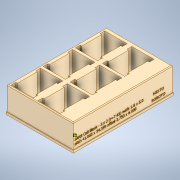
# Autodesk Inventor part: BlockTray_parameterized
Saved by Autodesk Inventor 2020 (Build 240168000, 168)
## iProperties
Created: 2019-12-05
Part Number: BlockTray_parameterized
Material: PC/ABS Plastic
Document SubType Name: Modeling
Designer: pab2
Density: 0.357273 g/cm^3
Appearance: Smooth - Off-White
Author: pab2
Autodesk Inventor part; units mm, degrees
(part 1 of 3)
ref_plane "YZ Plane" through (0, 0, 0) normal (1, 0, 0) x (0, 1, 0)
ref_plane "XZ Plane" through (0, 0, 0) normal (0, 1, 0) x (-1, 0, 0)
ref_plane "XY Plane" through (0, 0, 0) normal (0, 0, 1) x (1, 0, 0)
sketch "Sketch1" plane through (0, 0, 0) normal (0, 1, 0) x (-1, 0, 0)
  line L0 (0, 0) -> (-85.5, 0)
  line L1 (-85.5, 0) -> (-85.5, -127.75)
  line L2 (-85.5, -127.75) -> (0, -127.75)
  line L3 (0, -127.75) -> (0, 0)
  dimension "BaseW" = 85.5
  dimension "BaseL" = 127.75
  constraints: 8 end point, 2 parallel, 1 horizontal, 1 perpendicular
  measures "BaseW" distance of L2.end L1.end
  measures "BaseL" distance of L1.end L0.end
extrude "Extrusion1" add sketch "Sketch1" along normal blind 3
sketch "Sketch2" plane through (0, 3, 0) normal (0, 1, 0) x (1, 0, 0)
  line L0 (0, 127.75) -> (0, 0) projected
  line L1 (0, 0) -> (0.7071, 0.7071)
  line L2 (0, 0) -> (1, 0) construction
  line L3 (85.5, 127.75) -> (0, 127.75) projected
  line L4 (85.5, 127.75) -> (84.7929, 127.0429)
  line L5 (85.5, 127.75) -> (86.5, 127.75) construction
  line L6 (0.7071, 0.7071) -> (84.7929, 0.7071)
  line L7 (84.7929, 0.7071) -> (84.7929, 127.0429)
  line L8 (84.7929, 127.0429) -> (0.7071, 127.0429)
  line L9 (0.7071, 127.0429) -> (0.7071, 0.7071)
  dimension "RimOffset" = 1
  dimension "d5" = 45
  dimension "d6" = 1
  dimension "d7" = 225
  constraints: 16 end point, 3 horizontal, 2 equal length, 2 parallel, 1 perpendicular
  measures "RimOffset" distance of L0.end L1.end
  measures "d5" angle of L2 L1
  measures "d6" distance of L3.start L4.end
extrude "Extrusion2" add sketch "Sketch2" along normal blind 30 contours L9 L8 L7 L6
sketch "Sketch4" plane through (0, 33, 0) normal (0, 1, 0) x (1, 0, 0)
  line L0 (0.7071, 0.7071) -> (17.8022, 0.7071) construction
  line L1 (0.7071, 0.7071) -> (84.7929, 0.7071) projected
  line L2 (0.7071, 0.7071) -> (5.7071, 0.7071)
  line L3 (84.7929, 0.7071) -> (0.7071, 0.7071) projected
  line L4 (5.7071, 0.7071) -> (5.7071, 2.4571)
  line L5 (5.7071, 2.4571) -> (30.0657, 2.4571)
  line L6 (30.0657, 2.4571) -> (30.0657, 39.9602)
  line L7 (30.0657, 39.9602) -> (5.7071, 39.9602)
  line L8 (5.7071, 39.9602) -> (5.7071, 2.4571)
  line L9 (30.0657, 39.9602) -> (32.0657, 39.9602)
  line L10 (32.0657, 39.9602) -> (32.0657, 33.9602)
  line L11 (32.0657, 33.9602) -> (30.0657, 33.9602)
  line L12 (30.0657, 33.9602) -> (30.0657, 39.9602)
  line L13 (30.0657, 2.4571) -> (32.0657, 2.4571)
  line L14 (32.0657, 2.4571) -> (32.0657, 8.4571)
  line L15 (32.0657, 8.4571) -> (30.0657, 8.4571)
  line L16 (30.0657, 8.4571) -> (30.0657, 2.4571)
  line L17 (5.7071, 39.9602) -> (3.7071, 39.9602)
  line L18 (3.7071, 39.9602) -> (3.7071, 33.9602)
  line L19 (3.7071, 33.9602) -> (5.7071, 33.9602)
  line L20 (5.7071, 33.9602) -> (5.7071, 39.9602)
  line L21 (5.7071, 2.4571) -> (3.7071, 2.4571)
  line L22 (3.7071, 2.4571) -> (3.7071, 8.4571)
  line L23 (3.7071, 8.4571) -> (5.7071, 8.4571)
  line L24 (5.7071, 8.4571) -> (5.7071, 2.4571)
  point P0 (0, 0)
  point P1 (5.7071, 33.9602)
  point P2 (5.7071, 8.4571)
  point P3 (30.0657, 8.4571)
  dimension "d51" = 5
  dimension "d63" = 1.75
  dimension "d64" = 24.3586
  dimension "d65" = 37.5031
  dimension "ScrewProtrusionD" = 2
  dimension "ScrewProtrusionL" = 6
  dimension "d68" = 2
  dimension "d69" = 6
  dimension "d70" = 2
  dimension "d71" = 6
  dimension "d72" = 2
  dimension "d73" = 6
  constraints: 46 end point, 10 parallel, 6 horizontal, 6 perpendicular, 1 point on line
  measures "d51" distance of L0.start L2.end
  measures "d63" distance of L2.end L4.end
  measures "d64" distance of L7.end L6.end
  measures "d65" distance of L6.end L5.end
  measures "ScrewProtrusionD" distance of L10.end L11.end
  measures "ScrewProtrusionL" distance of L9.end L10.end
  measures "d68" distance of L15.end L14.end
  measures "d69" distance of L14.end L13.end
  measures "d70" distance of L19.end L18.end
  measures "d71" distance of L18.end L17.end
  measures "d72" distance of L22.end L23.end
  measures "d73" distance of L21.end L22.end
extrude "Extrusion3" cut sketch "Sketch4" against normal blind 30 from surface at 0
fillet "Fillet1" radius 1 4 edges at (42.75, 33, -0.7071) (84.7929, 33, -63.875) (0.7071, 33, -63.875) (42.75, 33, -127.0429)
pattern_linear "Rectangular Pattern2" count 2 spacing 34.3586 along (1, 0, 0) count 3 spacing 41.0031 along (0, 0, -1) of "Extrusion3"
sketch "Sketch5" plane through (84.7929, 3, -0.7071) normal (1, 0, 0) x (0, 0, -1)
  line L0 (1.5806, 11.976) -> (92.4463, 11.976) construction
  line L1 (92.4463, 11.976) -> (92.4463, 1.5433) construction
  line L2 (92.4463, 1.5433) -> (1.5806, 1.5433) construction
  line L3 (1.5806, 1.5433) -> (1.5806, 11.976) construction
  line L4 (95.1386, 13.0698) -> (121.8935, 13.0698) construction
  line L5 (121.8935, 13.0698) -> (121.8935, 1.4591) construction
  line L6 (121.8935, 1.4591) -> (95.1386, 1.4591) construction
  line L7 (95.1386, 1.4591) -> (95.1386, 13.0698) construction
  spline S0 degree 2 poles (2.7391, 8.7378) (2.4081, 8.7378) (1.9437, 8.8761) (1.7387, 8.9749) knots 0 0 0 1 2 2 2
  line L8 (1.7387, 8.9749) -> (1.7387, 9.4838)
  line L9 (1.7387, 9.4838) -> (1.7683, 9.4838)
  spline S1 degree 2 poles (1.7683, 9.4838) (1.9684, 9.296) (2.4748, 9.0886) (2.7094, 9.0886) knots 0 0 0 1 2 2 2
  spline S2 degree 2 poles (2.7094, 9.0886) (3.0453, 9.0886) (3.3887, 9.3677) (3.3887, 9.5974) knots 0 0 0 1 2 2 2
  spline S3 degree 2 poles (3.3887, 9.5974) (3.3887, 9.7802) (3.2084, 10.0074) (3.0132, 10.0642) knots 0 0 0 1 2 2 2
  spline S4 degree 2 poles (3.0132, 10.0642) (2.8724, 10.1037) (2.6378, 10.1581) (2.4624, 10.2025) knots 0 0 0 1 2 2 2
  spline S5 degree 2 poles (2.4624, 10.2025) (2.3043, 10.2445) (2.0549, 10.3705) (1.9585, 10.4718) knots 0 0 0 1 2 2 2
  spline S6 degree 2 poles (1.9585, 10.4718) (1.8647, 10.573) (1.7609, 10.8447) (1.7609, 11.0226) knots 0 0 0 1 2 2 2
  spline S7 degree 2 poles (1.7609, 11.0226) (1.7609, 11.3931) (2.3389, 11.8945) (2.786, 11.8945) knots 0 0 0 1 2 2 2
  spline S8 degree 2 poles (2.786, 11.8945) (3.0429, 11.8945) (3.4973, 11.7932) (3.6925, 11.6969) knots 0 0 0 1 2 2 2
  line L10 (3.6925, 11.6969) -> (3.6925, 11.2128)
  line L11 (3.6925, 11.2128) -> (3.6628, 11.2128)
  spline S9 degree 2 poles (3.6628, 11.2128) (3.5171, 11.3462) (3.0626, 11.5438) (2.8132, 11.5438) knots 0 0 0 1 2 2 2
  spline S10 degree 2 poles (2.8132, 11.5438) (2.5316, 11.5438) (2.1833, 11.2795) (2.1833, 11.0646) knots 0 0 0 1 2 2 2
  spline S11 degree 2 poles (2.1833, 11.0646) (2.1833, 10.8719) (2.3883, 10.6422) (2.581, 10.5903) knots 0 0 0 1 2 2 2
  spline S12 degree 2 poles (2.581, 10.5903) (2.7094, 10.5558) (3.0824, 10.4668) (3.2059, 10.4298) knots 0 0 0 1 2 2 2
  spline S13 degree 2 poles (3.2059, 10.4298) (3.5196, 10.3335) (3.811, 9.9457) (3.811, 9.6616) knots 0 0 0 1 2 2 2
  spline S14 degree 2 poles (3.811, 9.6616) (3.811, 9.4813) (3.6653, 9.1355) (3.5344, 9.0145) knots 0 0 0 1 2 2 2
  spline S15 degree 2 poles (3.5344, 9.0145) (3.3887, 8.8811) (3.0182, 8.7378) (2.7391, 8.7378) knots 0 0 0 1 2 2 2
  line L12 (3.895, 8.7922) -> (4.9225, 11.8402)
  line L13 (4.9225, 11.8402) -> (5.4215, 11.8402)
  line L14 (5.4215, 11.8402) -> (6.449, 8.7922)
  line L15 (6.449, 8.7922) -> (6.0217, 8.7922)
  line L16 (6.0217, 8.7922) -> (5.7451, 9.6443)
  line L17 (5.7451, 9.6443) -> (4.5817, 9.6443)
  line L18 (4.5817, 9.6443) -> (4.305, 8.7922)
  line L19 (4.305, 8.7922) -> (3.895, 8.7922)
  line L20 (5.6339, 9.9901) -> (5.1621, 11.4252)
  line L21 (5.1621, 11.4252) -> (4.6928, 9.9901)
  line L22 (4.6928, 9.9901) -> (5.6339, 9.9901)
  line L23 (8.919, 8.7922) -> (8.4646, 8.7922)
  line L24 (8.4646, 8.7922) -> (7.1159, 11.4203)
  line L25 (7.1159, 11.4203) -> (7.1159, 8.7922)
  line L26 (7.1159, 8.7922) -> (6.738, 8.7922)
  line L27 (6.738, 8.7922) -> (6.738, 11.8402)
  line L28 (6.738, 11.8402) -> (7.3135, 11.8402)
  line L29 (7.3135, 11.8402) -> (8.5411, 9.427)
  line L30 (8.5411, 9.427) -> (8.5411, 11.8402)
  line L31 (8.5411, 11.8402) -> (8.919, 11.8402)
  line L32 (8.919, 11.8402) -> (8.919, 8.7922)
  spline S16 degree 2 poles (10.3862, 8.7378) (10.0552, 8.7378) (9.5909, 8.8761) (9.3859, 8.9749) knots 0 0 0 1 2 2 2
  line L33 (9.3859, 8.9749) -> (9.3859, 9.4838)
  line L34 (9.3859, 9.4838) -> (9.4155, 9.4838)
  spline S17 degree 2 poles (9.4155, 9.4838) (9.6156, 9.296) (10.1219, 9.0886) (10.3566, 9.0886) knots 0 0 0 1 2 2 2
  spline S18 degree 2 poles (10.3566, 9.0886) (10.6925, 9.0886) (11.0358, 9.3677) (11.0358, 9.5974) knots 0 0 0 1 2 2 2
  spline S19 degree 2 poles (11.0358, 9.5974) (11.0358, 9.7802) (10.8555, 10.0074) (10.6604, 10.0642) knots 0 0 0 1 2 2 2
  spline S20 degree 2 poles (10.6604, 10.0642) (10.5196, 10.1037) (10.285, 10.1581) (10.1096, 10.2025) knots 0 0 0 1 2 2 2
  spline S21 degree 2 poles (10.1096, 10.2025) (9.9515, 10.2445) (9.702, 10.3705) (9.6057, 10.4718) knots 0 0 0 1 2 2 2
  spline S22 degree 2 poles (9.6057, 10.4718) (9.5118, 10.573) (9.4081, 10.8447) (9.4081, 11.0226) knots 0 0 0 1 2 2 2
  spline S23 degree 2 poles (9.4081, 11.0226) (9.4081, 11.3931) (9.9861, 11.8945) (10.4332, 11.8945) knots 0 0 0 1 2 2 2
  spline S24 degree 2 poles (10.4332, 11.8945) (10.69, 11.8945) (11.1445, 11.7932) (11.3396, 11.6969) knots 0 0 0 1 2 2 2
  line L35 (11.3396, 11.6969) -> (11.3396, 11.2128)
  line L36 (11.3396, 11.2128) -> (11.31, 11.2128)
  spline S25 degree 2 poles (11.31, 11.2128) (11.1643, 11.3462) (10.7098, 11.5438) (10.4603, 11.5438) knots 0 0 0 1 2 2 2
  spline S26 degree 2 poles (10.4603, 11.5438) (10.1787, 11.5438) (9.8305, 11.2795) (9.8305, 11.0646) knots 0 0 0 1 2 2 2
  spline S27 degree 2 poles (9.8305, 11.0646) (9.8305, 10.8719) (10.0355, 10.6422) (10.2281, 10.5903) knots 0 0 0 1 2 2 2
  spline S28 degree 2 poles (10.2281, 10.5903) (10.3566, 10.5558) (10.7296, 10.4668) (10.8531, 10.4298) knots 0 0 0 1 2 2 2
  spline S29 degree 2 poles (10.8531, 10.4298) (11.1667, 10.3335) (11.4582, 9.9457) (11.4582, 9.6616) knots 0 0 0 1 2 2 2
  spline S30 degree 2 poles (11.4582, 9.6616) (11.4582, 9.4813) (11.3125, 9.1355) (11.1816, 9.0145) knots 0 0 0 1 2 2 2
  spline S31 degree 2 poles (11.1816, 9.0145) (11.0358, 8.8811) (10.6653, 8.7378) (10.3862, 8.7378) knots 0 0 0 1 2 2 2
  spline S32 degree 2 poles (14.3704, 8.7378) (14.074, 8.7378) (13.5725, 8.9379) (13.3898, 9.138) knots 0 0 0 1 2 2 2
  spline S33 degree 2 poles (13.3898, 9.138) (13.207, 9.3356) (13.0069, 9.9284) (13.0069, 10.3137) knots 0 0 0 1 2 2 2
  spline S34 degree 2 poles (13.0069, 10.3137) (13.0069, 10.6965) (13.202, 11.2646) (13.3873, 11.4746) knots 0 0 0 1 2 2 2
  spline S35 degree 2 poles (13.3873, 11.4746) (13.5701, 11.6796) (14.069, 11.8945) (14.3778, 11.8945) knots 0 0 0 1 2 2 2
  spline S36 degree 2 poles (14.3778, 11.8945) (14.5309, 11.8945) (14.8001, 11.85) (14.9138, 11.8155) knots 0 0 0 1 2 2 2
  spline S37 degree 2 poles (14.9138, 11.8155) (15.0126, 11.7834) (15.2176, 11.692) (15.3188, 11.6376) knots 0 0 0 1 2 2 2
  line L37 (15.3188, 11.6376) -> (15.3188, 11.1486)
  line L38 (15.3188, 11.1486) -> (15.2867, 11.1486)
  spline S38 degree 2 poles (15.2867, 11.1486) (15.2324, 11.198) (15.0644, 11.3363) (14.9434, 11.403) knots 0 0 0 1 2 2 2
  spline S39 degree 2 poles (14.9434, 11.403) (14.8273, 11.4672) (14.5531, 11.5487) (14.3753, 11.5487) knots 0 0 0 1 2 2 2
  spline S40 degree 2 poles (14.3753, 11.5487) (14.1802, 11.5487) (13.8319, 11.3881) (13.701, 11.235) knots 0 0 0 1 2 2 2
  spline S41 degree 2 poles (13.701, 11.235) (13.5725, 11.0794) (13.4293, 10.6076) (13.4293, 10.3137) knots 0 0 0 1 2 2 2
  spline S42 degree 2 poles (13.4293, 10.3137) (13.4293, 10) (13.58, 9.548) (13.7109, 9.3924) knots 0 0 0 1 2 2 2
  spline S43 degree 2 poles (13.7109, 9.3924) (13.8393, 9.2417) (14.1826, 9.0886) (14.3753, 9.0886) knots 0 0 0 1 2 2 2
  spline S44 degree 2 poles (14.3753, 9.0886) (14.5507, 9.0886) (14.8495, 9.175) (14.9656, 9.2392) knots 0 0 0 1 2 2 2
  spline S45 degree 2 poles (14.9656, 9.2392) (15.0768, 9.3035) (15.2423, 9.4368) (15.2892, 9.4838) knots 0 0 0 1 2 2 2
  line L39 (15.2892, 9.4838) -> (15.3188, 9.4838)
  line L40 (15.3188, 9.4838) -> (15.3188, 8.9996)
  spline S46 degree 2 poles (15.3188, 8.9996) (15.2176, 8.9527) (15.0397, 8.8663) (14.9138, 8.8267) knots 0 0 0 1 2 2 2
  spline S47 degree 2 poles (14.9138, 8.8267) (14.7804, 8.7823) (14.5531, 8.7378) (14.3704, 8.7378) knots 0 0 0 1 2 2 2
  spline S48 degree 2 poles (16.6601, 8.7403) (16.1117, 8.7403) (15.509, 9.3553) (15.509, 9.9234) knots 0 0 0 1 2 2 2
  spline S49 degree 2 poles (15.509, 9.9234) (15.509, 10.4817) (16.0944, 11.1436) (16.5662, 11.1436) knots 0 0 0 1 2 2 2
  spline S50 degree 2 poles (16.5662, 11.1436) (16.7786, 11.1436) (17.1071, 11.0201) (17.2282, 10.8892) knots 0 0 0 1 2 2 2
  spline S51 degree 2 poles (17.2282, 10.8892) (17.3517, 10.7583) (17.4826, 10.3804) (17.4826, 10.1062) knots 0 0 0 1 2 2 2
  line L41 (17.4826, 10.1062) -> (17.4826, 9.8963)
  line L42 (17.4826, 9.8963) -> (15.8993, 9.8963)
  spline S52 degree 2 poles (15.8993, 9.8963) (15.8993, 9.4986) (16.2994, 9.0762) (16.6551, 9.0762) knots 0 0 0 1 2 2 2
  spline S53 degree 2 poles (16.6551, 9.0762) (16.7811, 9.0762) (17.0256, 9.133) (17.1244, 9.1775) knots 0 0 0 1 2 2 2
  spline S54 degree 2 poles (17.1244, 9.1775) (17.2282, 9.2269) (17.3714, 9.3133) (17.4184, 9.3529) knots 0 0 0 1 2 2 2
  line L43 (17.4184, 9.3529) -> (17.4406, 9.3529)
  line L44 (17.4406, 9.3529) -> (17.4406, 8.933)
  spline S55 degree 2 poles (17.4406, 8.933) (17.3739, 8.9058) (17.1714, 8.8267) (17.0923, 8.8045) knots 0 0 0 1 2 2 2
  spline S56 degree 2 poles (17.0923, 8.8045) (16.9812, 8.7724) (16.7984, 8.7403) (16.6601, 8.7403) knots 0 0 0 1 2 2 2
  spline S57 degree 2 poles (17.1071, 10.1902) (17.1022, 10.3458) (17.038, 10.573) (16.9762, 10.6496) knots 0 0 0 1 2 2 2
  spline S58 degree 2 poles (16.9762, 10.6496) (16.9095, 10.7361) (16.6996, 10.8275) (16.544, 10.8275) knots 0 0 0 1 2 2 2
  spline S59 degree 2 poles (16.544, 10.8275) (16.3908, 10.8275) (16.1759, 10.7361) (16.087, 10.6471) knots 0 0 0 1 2 2 2
  spline S60 degree 2 poles (16.087, 10.6471) (16.0006, 10.5558) (15.9116, 10.3359) (15.8993, 10.1902) knots 0 0 0 1 2 2 2
  line L45 (15.8993, 10.1902) -> (17.1071, 10.1902)
  line L46 (18.2656, 8.7922) -> (17.8803, 8.7922)
  line L47 (17.8803, 8.7922) -> (17.8803, 11.976)
  line L48 (17.8803, 11.976) -> (18.2656, 11.976)
  line L49 (18.2656, 11.976) -> (18.2656, 8.7922)
  line L50 (19.2239, 8.7922) -> (18.8386, 8.7922)
  line L51 (18.8386, 8.7922) -> (18.8386, 11.976)
  line L52 (18.8386, 11.976) -> (19.2239, 11.976)
  line L53 (19.2239, 11.976) -> (19.2239, 8.7922)
  spline S61 degree 2 poles (23.1957, 9.7283) (23.1957, 9.5011) (23.0228, 9.1528) (22.8796, 9.0392) knots 0 0 0 1 2 2 2
  spline S62 degree 2 poles (22.8796, 9.0392) (22.7067, 8.9058) (22.3139, 8.7922) (22.0027, 8.7922) knots 0 0 0 1 2 2 2
  line L54 (22.0027, 8.7922) -> (21.1283, 8.7922)
  line L55 (21.1283, 8.7922) -> (21.1283, 11.8402)
  line L56 (21.1283, 11.8402) -> (21.936, 11.8402)
  spline S63 degree 2 poles (21.936, 11.8402) (22.2621, 11.8402) (22.5881, 11.7982) (22.7363, 11.7167) knots 0 0 0 1 2 2 2
  spline S64 degree 2 poles (22.7363, 11.7167) (22.9018, 11.6302) (23.0525, 11.3462) (23.0525, 11.1535) knots 0 0 0 1 2 2 2
  spline S65 degree 2 poles (23.0525, 11.1535) (23.0525, 10.9386) (22.8252, 10.5977) (22.6252, 10.5014) knots 0 0 0 1 2 2 2
  line L57 (22.6252, 10.5014) -> (22.6252, 10.4866)
  spline S66 degree 2 poles (22.6252, 10.4866) (22.8969, 10.4125) (23.1957, 10.0198) (23.1957, 9.7283) knots 0 0 0 1 2 2 2
  spline S67 degree 2 poles (22.7734, 9.711) (22.7734, 9.8839) (22.6746, 10.1062) (22.5264, 10.1853) knots 0 0 0 1 2 2 2
  spline S68 degree 2 poles (22.5264, 10.1853) (22.43, 10.2347) (22.2028, 10.2643) (21.9928, 10.2643) knots 0 0 0 1 2 2 2
  line L58 (21.9928, 10.2643) -> (21.5334, 10.2643)
  line L59 (21.5334, 10.2643) -> (21.5334, 9.138)
  line L60 (21.5334, 9.138) -> (21.8619, 9.138)
  spline S69 degree 2 poles (21.8619, 9.138) (22.1287, 9.138) (22.435, 9.1874) (22.5535, 9.2664) knots 0 0 0 1 2 2 2
  spline S70 degree 2 poles (22.5535, 9.2664) (22.6671, 9.3479) (22.7734, 9.5505) (22.7734, 9.711) knots 0 0 0 1 2 2 2
  spline S71 degree 2 poles (22.6301, 11.0967) (22.6301, 11.2054) (22.556, 11.3684) (22.4745, 11.4153) knots 0 0 0 1 2 2 2
  spline S72 degree 2 poles (22.4745, 11.4153) (22.3757, 11.4697) (22.1361, 11.4944) (21.9212, 11.4944) knots 0 0 0 1 2 2 2
  line L61 (21.9212, 11.4944) -> (21.5334, 11.4944)
  line L62 (21.5334, 11.4944) -> (21.5334, 10.6027)
  line L63 (21.5334, 10.6027) -> (21.9928, 10.6027)
  spline S73 degree 2 poles (21.9928, 10.6027) (22.183, 10.6027) (22.3633, 10.6422) (22.4597, 10.704) knots 0 0 0 1 2 2 2
  spline S74 degree 2 poles (22.4597, 10.704) (22.5535, 10.7632) (22.6301, 10.9534) (22.6301, 11.0967) knots 0 0 0 1 2 2 2
  line L64 (23.9614, 8.7922) -> (23.5761, 8.7922)
  line L65 (23.5761, 8.7922) -> (23.5761, 11.976)
  line L66 (23.5761, 11.976) -> (23.9614, 11.976)
  line L67 (23.9614, 11.976) -> (23.9614, 8.7922)
  spline S75 degree 2 poles (26.4067, 9.9358) (26.4067, 9.3578) (25.851, 8.7279) (25.3866, 8.7279) knots 0 0 0 1 2 2 2
  spline S76 degree 2 poles (25.3866, 8.7279) (24.9099, 8.7279) (24.364, 9.3776) (24.364, 9.9358) knots 0 0 0 1 2 2 2
  spline S77 degree 2 poles (24.364, 9.9358) (24.364, 10.5088) (24.9272, 11.1436) (25.3866, 11.1436) knots 0 0 0 1 2 2 2
  spline S78 degree 2 poles (25.3866, 11.1436) (25.851, 11.1436) (26.4067, 10.5113) (26.4067, 9.9358) knots 0 0 0 1 2 2 2
  spline S79 degree 2 poles (26.0091, 9.9358) (26.0091, 10.3804) (25.6855, 10.8126) (25.3866, 10.8126) knots 0 0 0 1 2 2 2
  spline S80 degree 2 poles (25.3866, 10.8126) (25.0878, 10.8126) (24.7617, 10.3804) (24.7617, 9.9358) knots 0 0 0 1 2 2 2
  spline S81 degree 2 poles (24.7617, 9.9358) (24.7617, 9.5035) (25.0878, 9.0589) (25.3866, 9.0589) knots 0 0 0 1 2 2 2
  spline S82 degree 2 poles (25.3866, 9.0589) (25.683, 9.0589) (26.0091, 9.4961) (26.0091, 9.9358) knots 0 0 0 1 2 2 2
  spline S83 degree 2 poles (27.7109, 8.7403) (27.4738, 8.7403) (27.0811, 8.886) (26.9403, 9.0342) knots 0 0 0 1 2 2 2
  spline S84 degree 2 poles (26.9403, 9.0342) (26.7995, 9.18) (26.6439, 9.6295) (26.6439, 9.9308) knots 0 0 0 1 2 2 2
  spline S85 degree 2 poles (26.6439, 9.9308) (26.6439, 10.2322) (26.8044, 10.6718) (26.9403, 10.82) knots 0 0 0 1 2 2 2
  spline S86 degree 2 poles (26.9403, 10.82) (27.0761, 10.9707) (27.4787, 11.1313) (27.7109, 11.1313) knots 0 0 0 1 2 2 2
  spline S87 degree 2 poles (27.7109, 11.1313) (27.8986, 11.1313) (28.2494, 11.0251) (28.3852, 10.9559) knots 0 0 0 1 2 2 2
  line L68 (28.3852, 10.9559) -> (28.3852, 10.5236)
  line L69 (28.3852, 10.5236) -> (28.363, 10.5236)
  spline S88 degree 2 poles (28.363, 10.5236) (28.321, 10.5582) (28.1926, 10.6471) (28.1012, 10.6941) knots 0 0 0 1 2 2 2
  spline S89 degree 2 poles (28.1012, 10.6941) (28.0197, 10.7336) (27.8023, 10.7953) (27.7035, 10.7953) knots 0 0 0 1 2 2 2
  spline S90 degree 2 poles (27.7035, 10.7953) (27.4046, 10.7953) (27.0415, 10.3433) (27.0415, 9.9308) knots 0 0 0 1 2 2 2
  spline S91 degree 2 poles (27.0415, 9.9308) (27.0415, 9.5282) (27.3923, 9.0762) (27.7035, 9.0762) knots 0 0 0 1 2 2 2
  spline S92 degree 2 poles (27.7035, 9.0762) (27.8912, 9.0762) (28.2321, 9.2318) (28.363, 9.3529) knots 0 0 0 1 2 2 2
  line L70 (28.363, 9.3529) -> (28.3852, 9.3529)
  line L71 (28.3852, 9.3529) -> (28.3852, 8.9206)
  spline S93 degree 2 poles (28.3852, 8.9206) (28.3284, 8.8934) (28.1555, 8.8169) (28.0864, 8.7996) knots 0 0 0 1 2 2 2
  spline S94 degree 2 poles (28.0864, 8.7996) (27.9876, 8.7699) (27.8319, 8.7403) (27.7109, 8.7403) knots 0 0 0 1 2 2 2
  line L72 (30.6305, 8.7922) -> (30.1241, 8.7922)
  line L73 (30.1241, 8.7922) -> (29.2744, 9.8963)
  line L74 (29.2744, 9.8963) -> (29.1213, 9.7481)
  line L75 (29.1213, 9.7481) -> (29.1213, 8.7922)
  line L76 (29.1213, 8.7922) -> (28.736, 8.7922)
  line L77 (28.736, 8.7922) -> (28.736, 11.976)
  line L78 (28.736, 11.976) -> (29.1213, 11.976)
  line L79 (29.1213, 11.976) -> (29.1213, 10.1136)
  line L80 (29.1213, 10.1136) -> (30.0253, 11.0794)
  line L81 (30.0253, 11.0794) -> (30.5045, 11.0794)
  line L82 (30.5045, 11.0794) -> (29.5659, 10.1235)
  line L83 (29.5659, 10.1235) -> (30.6305, 8.7922)
  line L84 (33.1919, 9.9407) -> (32.0384, 9.9407)
  line L85 (32.0384, 9.9407) -> (32.0384, 10.3112)
  line L86 (32.0384, 10.3112) -> (33.1919, 10.3112)
  line L87 (33.1919, 10.3112) -> (33.1919, 9.9407)
  spline S95 degree 2 poles (35.7286, 11.5512) (35.6174, 11.5512) (35.3976, 11.4968) (35.2914, 11.4548) knots 0 0 0 1 2 2 2
  spline S96 degree 2 poles (35.2914, 11.4548) (35.1926, 11.4128) (35.0469, 11.3239) (34.9901, 11.2844) knots 0 0 0 1 2 2 2
  line L88 (34.9901, 11.2844) -> (34.9654, 11.2844)
  line L89 (34.9654, 11.2844) -> (34.9654, 11.7167)
  spline S97 degree 2 poles (34.9654, 11.7167) (35.0987, 11.7883) (35.5557, 11.9044) (35.7607, 11.9044) knots 0 0 0 1 2 2 2
  spline S98 degree 2 poles (35.7607, 11.9044) (35.9682, 11.9044) (36.2769, 11.8204) (36.4029, 11.7315) knots 0 0 0 1 2 2 2
  spline S99 degree 2 poles (36.4029, 11.7315) (36.5363, 11.6351) (36.6746, 11.356) (36.6746, 11.1683) knots 0 0 0 1 2 2 2
  spline S100 degree 2 poles (36.6746, 11.1683) (36.6746, 10.9164) (36.3436, 10.536) (36.1114, 10.4866) knots 0 0 0 1 2 2 2
  line L90 (36.1114, 10.4866) -> (36.1114, 10.457)
  spline S101 degree 2 poles (36.1114, 10.457) (36.2078, 10.4372) (36.4276, 10.3483) (36.5215, 10.2594) knots 0 0 0 1 2 2 2
  spline S102 degree 2 poles (36.5215, 10.2594) (36.6153, 10.1729) (36.7339, 9.8963) (36.7339, 9.6962) knots 0 0 0 1 2 2 2
  spline S103 degree 2 poles (36.7339, 9.6962) (36.7339, 9.4912) (36.5931, 9.1429) (36.4647, 9.0095) knots 0 0 0 1 2 2 2
  spline S104 degree 2 poles (36.4647, 9.0095) (36.3313, 8.8712) (35.9534, 8.7279) (35.7138, 8.7279) knots 0 0 0 1 2 2 2
  spline S105 degree 2 poles (35.7138, 8.7279) (35.4841, 8.7279) (35.0345, 8.8391) (34.8814, 8.9157) knots 0 0 0 1 2 2 2
  line L91 (34.8814, 8.9157) -> (34.8814, 9.3479)
  line L92 (34.8814, 9.3479) -> (34.911, 9.3479)
  spline S106 degree 2 poles (34.911, 9.3479) (35.0395, 9.2541) (35.4742, 9.0812) (35.6891, 9.0812) knots 0 0 0 1 2 2 2
  spline S107 degree 2 poles (35.6891, 9.0812) (35.815, 9.0812) (36.067, 9.1602) (36.151, 9.2516) knots 0 0 0 1 2 2 2
  spline S108 degree 2 poles (36.151, 9.2516) (36.2325, 9.343) (36.3189, 9.5603) (36.3189, 9.7258) knots 0 0 0 1 2 2 2
  spline S109 degree 2 poles (36.3189, 9.7258) (36.3189, 9.8913) (36.2226, 10.1062) (36.1361, 10.168) knots 0 0 0 1 2 2 2
  spline S110 degree 2 poles (36.1361, 10.168) (36.0497, 10.2297) (35.815, 10.2766) (35.6767, 10.2766) knots 0 0 0 1 2 2 2
  line L93 (35.6767, 10.2766) -> (35.5038, 10.2766)
  line L94 (35.5038, 10.2766) -> (35.5038, 10.615)
  line L95 (35.5038, 10.615) -> (35.6397, 10.615)
  spline S111 degree 2 poles (35.6397, 10.615) (35.9138, 10.615) (36.2596, 10.8769) (36.2596, 11.1263) knots 0 0 0 1 2 2 2
  spline S112 degree 2 poles (36.2596, 11.1263) (36.2596, 11.2424) (36.1707, 11.4079) (36.0991, 11.4573) knots 0 0 0 1 2 2 2
  spline S113 degree 2 poles (36.0991, 11.4573) (36.0225, 11.5092) (35.8348, 11.5512) (35.7286, 11.5512) knots 0 0 0 1 2 2 2
  line L96 (40.3352, 8.7922) -> (39.8634, 8.7922)
  line L97 (39.8634, 8.7922) -> (39.3076, 9.6517)
  line L98 (39.3076, 9.6517) -> (38.7371, 8.7922)
  line L99 (38.7371, 8.7922) -> (38.2999, 8.7922)
  line L100 (38.2999, 8.7922) -> (39.0928, 9.9259)
  line L101 (39.0928, 9.9259) -> (38.3073, 11.0794)
  line L102 (38.3073, 11.0794) -> (38.7791, 11.0794)
  line L103 (38.7791, 11.0794) -> (39.3323, 10.2272)
  line L104 (39.3323, 10.2272) -> (39.898, 11.0794)
  line L105 (39.898, 11.0794) -> (40.3352, 11.0794)
  line L106 (40.3352, 11.0794) -> (39.5472, 9.9506)
  line L107 (39.5472, 9.9506) -> (40.3352, 8.7922)
  line L108 (43.766, 8.7922) -> (41.8863, 8.7922)
  line L109 (41.8863, 8.7922) -> (41.8863, 9.2244)
  spline S114 degree 2 poles (41.8863, 9.2244) (42.0889, 9.4146) (42.4495, 9.7678) (42.6224, 9.958) knots 0 0 0 1 2 2 2
  spline S115 degree 2 poles (42.6224, 9.958) (42.9707, 10.3409) (43.2251, 10.8003) (43.2251, 11.0448) knots 0 0 0 1 2 2 2
  spline S116 degree 2 poles (43.2251, 11.0448) (43.2251, 11.1733) (43.146, 11.3659) (43.0744, 11.4277) knots 0 0 0 1 2 2 2
  spline S117 degree 2 poles (43.0744, 11.4277) (43.0028, 11.4894) (42.8151, 11.5512) (42.7014, 11.5512) knots 0 0 0 1 2 2 2
  spline S118 degree 2 poles (42.7014, 11.5512) (42.5928, 11.5512) (42.3705, 11.4968) (42.2692, 11.4548) knots 0 0 0 1 2 2 2
  spline S119 degree 2 poles (42.2692, 11.4548) (42.1827, 11.4203) (42.0222, 11.3215) (41.9728, 11.2869) knots 0 0 0 1 2 2 2
  line L110 (41.9728, 11.2869) -> (41.9506, 11.2869)
  line L111 (41.9506, 11.2869) -> (41.9506, 11.7216)
  spline S120 degree 2 poles (41.9506, 11.7216) (42.0765, 11.7834) (42.5285, 11.9044) (42.7311, 11.9044) knots 0 0 0 1 2 2 2
  spline S121 degree 2 poles (42.7311, 11.9044) (43.1584, 11.9044) (43.6401, 11.4524) (43.6401, 11.067) knots 0 0 0 1 2 2 2
  spline S122 degree 2 poles (43.6401, 11.067) (43.6401, 10.8867) (43.5561, 10.5854) (43.482, 10.457) knots 0 0 0 1 2 2 2
  spline S123 degree 2 poles (43.482, 10.457) (43.4079, 10.3236) (43.193, 10.0617) (43.0744, 9.9358) knots 0 0 0 1 2 2 2
  spline S124 degree 2 poles (43.0744, 9.9358) (42.8818, 9.7258) (42.41, 9.2763) (42.2692, 9.1454) knots 0 0 0 1 2 2 2
  line L112 (42.2692, 9.1454) -> (43.766, 9.1454)
  line L113 (43.766, 9.1454) -> (43.766, 8.7922)
  line L114 (46.7128, 7.9499) -> (46.2434, 7.9499)
  spline S125 degree 2 poles (46.2434, 7.9499) (45.8878, 8.3723) (45.4802, 9.3183) (45.4802, 9.9629) knots 0 0 0 1 2 2 2
  spline S126 degree 2 poles (45.4802, 9.9629) (45.4802, 10.5928) (45.8828, 11.5536) (46.2434, 11.976) knots 0 0 0 1 2 2 2
  line L115 (46.2434, 11.976) -> (46.7128, 11.976)
  line L116 (46.7128, 11.976) -> (46.7128, 11.9563)
  spline S127 degree 2 poles (46.7128, 11.9563) (46.5473, 11.8056) (46.2459, 11.4153) (46.1175, 11.156) knots 0 0 0 1 2 2 2
  spline S128 degree 2 poles (46.1175, 11.156) (45.994, 10.904) (45.8408, 10.2989) (45.8408, 9.9629) knots 0 0 0 1 2 2 2
  spline S129 degree 2 poles (45.8408, 9.9629) (45.8408, 9.6122) (45.989, 9.0318) (46.1175, 8.7699) knots 0 0 0 1 2 2 2
  spline S130 degree 2 poles (46.1175, 8.7699) (46.241, 8.518) (46.5547, 8.1104) (46.7128, 7.9696) knots 0 0 0 1 2 2 2
  line L117 (46.7128, 7.9696) -> (46.7128, 7.9499)
  line L118 (48.3578, 10.6669) -> (48.338, 10.6669)
  spline S131 degree 2 poles (48.338, 10.6669) (48.2936, 10.6793) (48.1972, 10.6842) (48.1305, 10.6842) knots 0 0 0 1 2 2 2
  spline S132 degree 2 poles (48.1305, 10.6842) (47.9749, 10.6842) (47.6686, 10.5483) (47.5303, 10.415) knots 0 0 0 1 2 2 2
  line L119 (47.5303, 10.415) -> (47.5303, 8.7922)
  line L120 (47.5303, 8.7922) -> (47.145, 8.7922)
  line L121 (47.145, 8.7922) -> (47.145, 11.0794)
  line L122 (47.145, 11.0794) -> (47.5303, 11.0794)
  line L123 (47.5303, 11.0794) -> (47.5303, 10.7385)
  spline S133 degree 2 poles (47.5303, 10.7385) (47.7403, 10.9263) (48.054, 11.0794) (48.2022, 11.0794) knots 0 0 0 1 2 2 2
  spline S134 degree 2 poles (48.2022, 11.0794) (48.2615, 11.0794) (48.3207, 11.0745) (48.3578, 11.067) knots 0 0 0 1 2 2 2
  line L124 (48.3578, 11.067) -> (48.3578, 10.6669)
  line L125 (51.0328, 9.5332) -> (48.7703, 9.5332)
  line L126 (48.7703, 9.5332) -> (48.7703, 9.8617)
  line L127 (48.7703, 9.8617) -> (51.0328, 9.8617)
  line L128 (51.0328, 9.8617) -> (51.0328, 9.5332)
  line L129 (51.0328, 10.3927) -> (48.7703, 10.3927)
  line L130 (48.7703, 10.3927) -> (48.7703, 10.7212)
  line L131 (48.7703, 10.7212) -> (51.0328, 10.7212)
  line L132 (51.0328, 10.7212) -> (51.0328, 10.3927)
  line L133 (53.5646, 11.3832) -> (52.2456, 8.7922)
  line L134 (52.2456, 8.7922) -> (51.8109, 8.7922)
  line L135 (51.8109, 8.7922) -> (53.204, 11.482)
  line L136 (53.204, 11.482) -> (51.6306, 11.482)
  line L137 (51.6306, 11.482) -> (51.6306, 11.8402)
  line L138 (51.6306, 11.8402) -> (53.5646, 11.8402)
  line L139 (53.5646, 11.8402) -> (53.5646, 11.3832)
  line L140 (54.5921, 8.7922) -> (54.103, 8.7922)
  line L141 (54.103, 8.7922) -> (54.103, 9.3751)
  line L142 (54.103, 9.3751) -> (54.5921, 9.3751)
  line L143 (54.5921, 9.3751) -> (54.5921, 8.7922)
  line L144 (57.1683, 9.8394) -> (56.8052, 9.8394)
  line L145 (56.8052, 9.8394) -> (56.8052, 8.7922)
  line L146 (56.8052, 8.7922) -> (56.4125, 8.7922)
  line L147 (56.4125, 8.7922) -> (56.4125, 9.8394)
  line L148 (56.4125, 9.8394) -> (55.0663, 9.8394)
  line L149 (55.0663, 9.8394) -> (55.0663, 10.2692)
  line L150 (55.0663, 10.2692) -> (56.4298, 11.8402)
  line L151 (56.4298, 11.8402) -> (56.8052, 11.8402)
  line L152 (56.8052, 11.8402) -> (56.8052, 10.168)
  line L153 (56.8052, 10.168) -> (57.1683, 10.168)
  line L154 (57.1683, 10.168) -> (57.1683, 9.8394)
  line L155 (56.4125, 10.168) -> (56.4125, 11.3585)
  line L156 (56.4125, 11.3585) -> (55.3874, 10.168)
  line L157 (55.3874, 10.168) -> (56.4125, 10.168)
  spline S135 degree 2 poles (58.3169, 11.5512) (58.2057, 11.5512) (57.9859, 11.4968) (57.8797, 11.4548) knots 0 0 0 1 2 2 2
  spline S136 degree 2 poles (57.8797, 11.4548) (57.7809, 11.4128) (57.6352, 11.3239) (57.5784, 11.2844) knots 0 0 0 1 2 2 2
  line L158 (57.5784, 11.2844) -> (57.5537, 11.2844)
  line L159 (57.5537, 11.2844) -> (57.5537, 11.7167)
  spline S137 degree 2 poles (57.5537, 11.7167) (57.687, 11.7883) (58.144, 11.9044) (58.349, 11.9044) knots 0 0 0 1 2 2 2
  spline S138 degree 2 poles (58.349, 11.9044) (58.5565, 11.9044) (58.8652, 11.8204) (58.9912, 11.7315) knots 0 0 0 1 2 2 2
  spline S139 degree 2 poles (58.9912, 11.7315) (59.1246, 11.6351) (59.2629, 11.356) (59.2629, 11.1683) knots 0 0 0 1 2 2 2
  spline S140 degree 2 poles (59.2629, 11.1683) (59.2629, 10.9164) (58.9319, 10.536) (58.6997, 10.4866) knots 0 0 0 1 2 2 2
  line L160 (58.6997, 10.4866) -> (58.6997, 10.457)
  spline S141 degree 2 poles (58.6997, 10.457) (58.7961, 10.4372) (59.0159, 10.3483) (59.1098, 10.2594) knots 0 0 0 1 2 2 2
  spline S142 degree 2 poles (59.1098, 10.2594) (59.2036, 10.1729) (59.3222, 9.8963) (59.3222, 9.6962) knots 0 0 0 1 2 2 2
  spline S143 degree 2 poles (59.3222, 9.6962) (59.3222, 9.4912) (59.1814, 9.1429) (59.053, 9.0095) knots 0 0 0 1 2 2 2
  spline S144 degree 2 poles (59.053, 9.0095) (58.9196, 8.8712) (58.5417, 8.7279) (58.3021, 8.7279) knots 0 0 0 1 2 2 2
  spline S145 degree 2 poles (58.3021, 8.7279) (58.0724, 8.7279) (57.6228, 8.8391) (57.4697, 8.9157) knots 0 0 0 1 2 2 2
  line L161 (57.4697, 8.9157) -> (57.4697, 9.3479)
  line L162 (57.4697, 9.3479) -> (57.4993, 9.3479)
  spline S146 degree 2 poles (57.4993, 9.3479) (57.6278, 9.2541) (58.0625, 9.0812) (58.2774, 9.0812) knots 0 0 0 1 2 2 2
  spline S147 degree 2 poles (58.2774, 9.0812) (58.4033, 9.0812) (58.6553, 9.1602) (58.7393, 9.2516) knots 0 0 0 1 2 2 2
  spline S148 degree 2 poles (58.7393, 9.2516) (58.8208, 9.343) (58.9072, 9.5603) (58.9072, 9.7258) knots 0 0 0 1 2 2 2
  spline S149 degree 2 poles (58.9072, 9.7258) (58.9072, 9.8913) (58.8109, 10.1062) (58.7244, 10.168) knots 0 0 0 1 2 2 2
  spline S150 degree 2 poles (58.7244, 10.168) (58.638, 10.2297) (58.4033, 10.2766) (58.265, 10.2766) knots 0 0 0 1 2 2 2
  line L163 (58.265, 10.2766) -> (58.0921, 10.2766)
  line L164 (58.0921, 10.2766) -> (58.0921, 10.615)
  line L165 (58.0921, 10.615) -> (58.228, 10.615)
  spline S151 degree 2 poles (58.228, 10.615) (58.5021, 10.615) (58.8479, 10.8769) (58.8479, 11.1263) knots 0 0 0 1 2 2 2
  spline S152 degree 2 poles (58.8479, 11.1263) (58.8479, 11.2424) (58.759, 11.4079) (58.6874, 11.4573) knots 0 0 0 1 2 2 2
  spline S153 degree 2 poles (58.6874, 11.4573) (58.6108, 11.5092) (58.4231, 11.5512) (58.3169, 11.5512) knots 0 0 0 1 2 2 2
  spline S154 degree 2 poles (60.945, 9.9629) (60.945, 9.3306) (60.5399, 8.3723) (60.1818, 7.9499) knots 0 0 0 1 2 2 2
  line L166 (60.1818, 7.9499) -> (59.7124, 7.9499)
  line L167 (59.7124, 7.9499) -> (59.7124, 7.9696)
  spline S155 degree 2 poles (59.7124, 7.9696) (59.8705, 8.1104) (60.1892, 8.5229) (60.3077, 8.7699) knots 0 0 0 1 2 2 2
  spline S156 degree 2 poles (60.3077, 8.7699) (60.4362, 9.0342) (60.5844, 9.6221) (60.5844, 9.9629) knots 0 0 0 1 2 2 2
  spline S157 degree 2 poles (60.5844, 9.9629) (60.5844, 10.3013) (60.4337, 10.9016) (60.3077, 11.156) knots 0 0 0 1 2 2 2
  spline S158 degree 2 poles (60.3077, 11.156) (60.1842, 11.4104) (59.8681, 11.8155) (59.7124, 11.9563) knots 0 0 0 1 2 2 2
  line L168 (59.7124, 11.9563) -> (59.7124, 11.976)
  line L169 (59.7124, 11.976) -> (60.1818, 11.976)
  spline S159 degree 2 poles (60.1818, 11.976) (60.5374, 11.5536) (60.945, 10.6002) (60.945, 9.9629) knots 0 0 0 1 2 2 2
  line L170 (65.5244, 11.0794) -> (64.9439, 8.7922)
  line L171 (64.9439, 8.7922) -> (64.5883, 8.7922)
  line L172 (64.5883, 8.7922) -> (64.03, 10.5558)
  line L173 (64.03, 10.5558) -> (63.4743, 8.7922)
  line L174 (63.4743, 8.7922) -> (63.1211, 8.7922)
  line L175 (63.1211, 8.7922) -> (62.5357, 11.0794)
  line L176 (62.5357, 11.0794) -> (62.9358, 11.0794)
  line L177 (62.9358, 11.0794) -> (63.3409, 9.3084)
  line L178 (63.3409, 9.3084) -> (63.8818, 11.0794)
  line L179 (63.8818, 11.0794) -> (64.2005, 11.0794)
  line L180 (64.2005, 11.0794) -> (64.7562, 9.3084)
  line L181 (64.7562, 9.3084) -> (65.1366, 11.0794)
  line L182 (65.1366, 11.0794) -> (65.5244, 11.0794)
  spline S160 degree 2 poles (67.1373, 9.0342) (67.0904, 8.9996) (66.9323, 8.8761) (66.8582, 8.8391) knots 0 0 0 1 2 2 2
  spline S161 degree 2 poles (66.8582, 8.8391) (66.7569, 8.7848) (66.5667, 8.7279) (66.3938, 8.7279) knots 0 0 0 1 2 2 2
  spline S162 degree 2 poles (66.3938, 8.7279) (66.2531, 8.7279) (65.9986, 8.8342) (65.9023, 8.9305) knots 0 0 0 1 2 2 2
  spline S163 degree 2 poles (65.9023, 8.9305) (65.8109, 9.0243) (65.6998, 9.301) (65.6998, 9.4541) knots 0 0 0 1 2 2 2
  spline S164 degree 2 poles (65.6998, 9.4541) (65.6998, 9.6912) (65.8998, 10.0272) (66.1172, 10.1235) knots 0 0 0 1 2 2 2
  spline S165 degree 2 poles (66.1172, 10.1235) (66.3099, 10.2124) (66.8335, 10.2791) (67.1373, 10.2964) knots 0 0 0 1 2 2 2
  line L183 (67.1373, 10.2964) -> (67.1373, 10.3705)
  spline S166 degree 2 poles (67.1373, 10.3705) (67.1373, 10.5039) (67.0558, 10.6694) (66.9817, 10.7163) knots 0 0 0 1 2 2 2
  spline S167 degree 2 poles (66.9817, 10.7163) (66.9076, 10.7632) (66.6952, 10.7929) (66.5816, 10.7929) knots 0 0 0 1 2 2 2
  spline S168 degree 2 poles (66.5816, 10.7929) (66.4482, 10.7929) (66.0876, 10.7138) (65.9072, 10.6373) knots 0 0 0 1 2 2 2
  line L184 (65.9072, 10.6373) -> (65.885, 10.6373)
  line L185 (65.885, 10.6373) -> (65.885, 11.03)
  spline S169 degree 2 poles (65.885, 11.03) (65.9912, 11.0596) (66.3889, 11.1337) (66.584, 11.1337) knots 0 0 0 1 2 2 2
  spline S170 degree 2 poles (66.584, 11.1337) (66.8212, 11.1337) (67.1447, 11.0596) (67.2732, 10.9633) knots 0 0 0 1 2 2 2
  spline S171 degree 2 poles (67.2732, 10.9633) (67.3991, 10.8694) (67.5226, 10.5706) (67.5226, 10.3557) knots 0 0 0 1 2 2 2
  line L186 (67.5226, 10.3557) -> (67.5226, 8.7922)
  line L187 (67.5226, 8.7922) -> (67.1373, 8.7922)
  line L188 (67.1373, 8.7922) -> (67.1373, 9.0342)
  line L189 (67.1373, 9.3553) -> (67.1373, 9.9901)
  spline S172 degree 2 poles (67.1373, 9.9901) (66.999, 9.9778) (66.5816, 9.9358) (66.4507, 9.8963) knots 0 0 0 1 2 2 2
  spline S173 degree 2 poles (66.4507, 9.8963) (66.2975, 9.8493) (66.0974, 9.6542) (66.0974, 9.4813) knots 0 0 0 1 2 2 2
  spline S174 degree 2 poles (66.0974, 9.4813) (66.0974, 9.2837) (66.3197, 9.0836) (66.5322, 9.0836) knots 0 0 0 1 2 2 2
  spline S175 degree 2 poles (66.5322, 9.0836) (66.7125, 9.0836) (67.0089, 9.2392) (67.1373, 9.3553) knots 0 0 0 1 2 2 2
  line L190 (68.4563, 8.7922) -> (68.071, 8.7922)
  line L191 (68.071, 8.7922) -> (68.071, 11.976)
  line L192 (68.071, 11.976) -> (68.4563, 11.976)
  line L193 (68.4563, 11.976) -> (68.4563, 8.7922)
  line L194 (69.4147, 8.7922) -> (69.0293, 8.7922)
  line L195 (69.0293, 8.7922) -> (69.0293, 11.976)
  line L196 (69.0293, 11.976) -> (69.4147, 11.976)
  line L197 (69.4147, 11.976) -> (69.4147, 8.7922)
  spline S176 degree 2 poles (70.5978, 8.7378) (70.3681, 8.7378) (69.9704, 8.8613) (69.8395, 8.9305) knots 0 0 0 1 2 2 2
  line L198 (69.8395, 8.9305) -> (69.8395, 9.3627)
  line L199 (69.8395, 9.3627) -> (69.8593, 9.3627)
  spline S177 degree 2 poles (69.8593, 9.3627) (69.9087, 9.3232) (70.0421, 9.2294) (70.1532, 9.1775) knots 0 0 0 1 2 2 2
  spline S178 degree 2 poles (70.1532, 9.1775) (70.2495, 9.1306) (70.4867, 9.0614) (70.6126, 9.0614) knots 0 0 0 1 2 2 2
  spline S179 degree 2 poles (70.6126, 9.0614) (70.704, 9.0614) (70.914, 9.1034) (70.9634, 9.138) knots 0 0 0 1 2 2 2
  spline S180 degree 2 poles (70.9634, 9.138) (71.035, 9.1849) (71.0992, 9.2911) (71.0992, 9.3998) knots 0 0 0 1 2 2 2
  spline S181 degree 2 poles (71.0992, 9.3998) (71.0992, 9.5356) (70.951, 9.6764) (70.7608, 9.7234) knots 0 0 0 1 2 2 2
  spline S182 degree 2 poles (70.7608, 9.7234) (70.6867, 9.7406) (70.4496, 9.79) (70.3483, 9.8172) knots 0 0 0 1 2 2 2
  spline S183 degree 2 poles (70.3483, 9.8172) (70.0865, 9.8938) (69.8494, 10.21) (69.8494, 10.4347) knots 0 0 0 1 2 2 2
  spline S184 degree 2 poles (69.8494, 10.4347) (69.8494, 10.7459) (70.3162, 11.1337) (70.7015, 11.1337) knots 0 0 0 1 2 2 2
  spline S185 degree 2 poles (70.7015, 11.1337) (70.8917, 11.1337) (71.2771, 11.0399) (71.408, 10.9682) knots 0 0 0 1 2 2 2
  line L200 (71.408, 10.9682) -> (71.408, 10.5558)
  line L201 (71.408, 10.5558) -> (71.3882, 10.5558)
  spline S186 degree 2 poles (71.3882, 10.5558) (71.24, 10.6743) (70.8794, 10.8102) (70.6941, 10.8102) knots 0 0 0 1 2 2 2
  spline S187 degree 2 poles (70.6941, 10.8102) (70.5039, 10.8102) (70.2421, 10.6496) (70.2421, 10.4891) knots 0 0 0 1 2 2 2
  spline S188 degree 2 poles (70.2421, 10.4891) (70.2421, 10.3433) (70.3977, 10.2025) (70.5706, 10.1581) knots 0 0 0 1 2 2 2
  spline S189 degree 2 poles (70.5706, 10.1581) (70.6546, 10.1358) (70.867, 10.0914) (70.9831, 10.0642) knots 0 0 0 1 2 2 2
  spline S190 degree 2 poles (70.9831, 10.0642) (71.2351, 10) (71.492, 9.7061) (71.492, 9.4517) knots 0 0 0 1 2 2 2
  spline S191 degree 2 poles (71.492, 9.4517) (71.492, 9.3035) (71.3759, 9.0416) (71.2622, 8.9453) knots 0 0 0 1 2 2 2
  spline S192 degree 2 poles (71.2622, 8.9453) (71.1412, 8.844) (70.8325, 8.7378) (70.5978, 8.7378) knots 0 0 0 1 2 2 2
  line L202 (74.8289, 8.7922) -> (73.342, 8.7922)
  line L203 (73.342, 8.7922) -> (73.342, 9.1034)
  line L204 (73.342, 9.1034) -> (73.8953, 9.1034)
  line L205 (73.8953, 9.1034) -> (73.8953, 11.1461)
  line L206 (73.8953, 11.1461) -> (73.342, 11.1461)
  line L207 (73.342, 11.1461) -> (73.342, 11.4252)
  spline S193 degree 2 poles (73.342, 11.4252) (73.6557, 11.4252) (73.9521, 11.603) (73.9719, 11.85) knots 0 0 0 1 2 2 2
  line L208 (73.9719, 11.85) -> (74.288, 11.85)
  line L209 (74.288, 11.85) -> (74.288, 9.1034)
  line L210 (74.288, 9.1034) -> (74.8289, 9.1034)
  line L211 (74.8289, 9.1034) -> (74.8289, 8.7922)
  line L212 (76.0442, 8.7922) -> (75.5551, 8.7922)
  line L213 (75.5551, 8.7922) -> (75.5551, 9.3751)
  line L214 (75.5551, 9.3751) -> (76.0442, 9.3751)
  line L215 (76.0442, 9.3751) -> (76.0442, 8.7922)
  spline S194 degree 2 poles (77.5805, 8.723) (77.3533, 8.723) (76.9803, 8.8589) (76.8494, 8.9848) knots 0 0 0 1 2 2 2
  spline S195 degree 2 poles (76.8494, 8.9848) (76.721, 9.1083) (76.5876, 9.4442) (76.5876, 9.6344) knots 0 0 0 1 2 2 2
  spline S196 degree 2 poles (76.5876, 9.6344) (76.5876, 9.8814) (76.8519, 10.2964) (77.1038, 10.4199) knots 0 0 0 1 2 2 2
  line L216 (77.1038, 10.4199) -> (77.1038, 10.4323)
  spline S197 degree 2 poles (77.1038, 10.4323) (76.8791, 10.5632) (76.6617, 10.8744) (76.6617, 11.1066) knots 0 0 0 1 2 2 2
  spline S198 degree 2 poles (76.6617, 11.1066) (76.6617, 11.4499) (77.1804, 11.9093) (77.5805, 11.9093) knots 0 0 0 1 2 2 2
  spline S199 degree 2 poles (77.5805, 11.9093) (77.9955, 11.9093) (78.4969, 11.4746) (78.4969, 11.1337) knots 0 0 0 1 2 2 2
  spline S200 degree 2 poles (78.4969, 11.1337) (78.4969, 10.9287) (78.2573, 10.5286) (78.0326, 10.415) knots 0 0 0 1 2 2 2
  line L217 (78.0326, 10.415) -> (78.0326, 10.4026)
  spline S201 degree 2 poles (78.0326, 10.4026) (78.2993, 10.2791) (78.5735, 9.9234) (78.5735, 9.6418) knots 0 0 0 1 2 2 2
  spline S202 degree 2 poles (78.5735, 9.6418) (78.5735, 9.2516) (78.0054, 8.723) (77.5805, 8.723) knots 0 0 0 1 2 2 2
  spline S203 degree 2 poles (78.1536, 9.6023) (78.1536, 9.79) (78.0054, 10.0123) (77.7954, 10.126) knots 0 0 0 1 2 2 2
  spline S204 degree 2 poles (77.7954, 10.126) (77.7263, 10.1655) (77.4941, 10.2569) (77.3484, 10.3162) knots 0 0 0 1 2 2 2
  spline S205 degree 2 poles (77.3484, 10.3162) (77.1804, 10.205) (77.0001, 9.874) (77.0001, 9.6641) knots 0 0 0 1 2 2 2
  spline S206 degree 2 poles (77.0001, 9.6641) (77.0001, 9.3874) (77.3335, 9.0268) (77.5855, 9.0268) knots 0 0 0 1 2 2 2
  spline S207 degree 2 poles (77.5855, 9.0268) (77.8424, 9.0268) (78.1536, 9.3356) (78.1536, 9.6023) knots 0 0 0 1 2 2 2
  spline S208 degree 2 poles (78.0968, 11.1288) (78.0968, 11.3338) (77.8226, 11.608) (77.5781, 11.608) knots 0 0 0 1 2 2 2
  spline S209 degree 2 poles (77.5781, 11.608) (77.3558, 11.608) (77.0717, 11.3634) (77.0717, 11.1535) knots 0 0 0 1 2 2 2
  spline S210 degree 2 poles (77.0717, 11.1535) (77.0717, 11.0028) (77.2175, 10.7929) (77.3632, 10.7089) knots 0 0 0 1 2 2 2
  spline S211 degree 2 poles (77.3632, 10.7089) (77.4249, 10.6743) (77.6868, 10.5533) (77.793, 10.5187) knots 0 0 0 1 2 2 2
  spline S212 degree 2 poles (77.793, 10.5187) (77.9708, 10.6546) (78.0968, 10.9435) (78.0968, 11.1288) knots 0 0 0 1 2 2 2
  line L218 (82.0883, 8.7922) -> (81.6166, 8.7922)
  line L219 (81.6166, 8.7922) -> (81.0608, 9.6517)
  line L220 (81.0608, 9.6517) -> (80.4902, 8.7922)
  line L221 (80.4902, 8.7922) -> (80.053, 8.7922)
  line L222 (80.053, 8.7922) -> (80.8459, 9.9259)
  line L223 (80.8459, 9.9259) -> (80.0604, 11.0794)
  line L224 (80.0604, 11.0794) -> (80.5322, 11.0794)
  line L225 (80.5322, 11.0794) -> (81.0855, 10.2272)
  line L226 (81.0855, 10.2272) -> (81.6511, 11.0794)
  line L227 (81.6511, 11.0794) -> (82.0883, 11.0794)
  line L228 (82.0883, 11.0794) -> (81.3004, 9.9506)
  line L229 (81.3004, 9.9506) -> (82.0883, 8.7922)
  spline S213 degree 2 poles (85.4871, 9.7604) (85.4871, 9.5406) (85.3463, 9.1651) (85.2178, 9.0268) knots 0 0 0 1 2 2 2
  spline S214 degree 2 poles (85.2178, 9.0268) (85.0894, 8.8885) (84.7065, 8.7279) (84.4694, 8.7279) knots 0 0 0 1 2 2 2
  spline S215 degree 2 poles (84.4694, 8.7279) (84.2521, 8.7279) (83.8272, 8.8243) (83.6716, 8.9008) knots 0 0 0 1 2 2 2
  line L230 (83.6716, 8.9008) -> (83.6716, 9.3331)
  line L231 (83.6716, 9.3331) -> (83.7012, 9.3331)
  spline S216 degree 2 poles (83.7012, 9.3331) (83.7482, 9.2985) (83.9235, 9.2096) (84.0298, 9.1701) knots 0 0 0 1 2 2 2
  spline S217 degree 2 poles (84.0298, 9.1701) (84.1508, 9.1281) (84.3509, 9.0812) (84.4768, 9.0812) knots 0 0 0 1 2 2 2
  spline S218 degree 2 poles (84.4768, 9.0812) (84.6003, 9.0812) (84.8325, 9.1701) (84.9165, 9.2664) knots 0 0 0 1 2 2 2
  spline S219 degree 2 poles (84.9165, 9.2664) (84.9931, 9.3578) (85.0721, 9.5999) (85.0721, 9.7629) knots 0 0 0 1 2 2 2
  spline S220 degree 2 poles (85.0721, 9.7629) (85.0721, 9.9259) (84.9832, 10.1334) (84.8992, 10.2025) knots 0 0 0 1 2 2 2
  spline S221 degree 2 poles (84.8992, 10.2025) (84.8128, 10.2791) (84.5559, 10.3433) (84.4003, 10.3433) knots 0 0 0 1 2 2 2
  spline S222 degree 2 poles (84.4003, 10.3433) (84.2323, 10.3433) (83.8988, 10.2915) (83.7976, 10.2692) knots 0 0 0 1 2 2 2
  line L232 (83.7976, 10.2692) -> (83.7976, 11.8402)
  line L233 (83.7976, 11.8402) -> (85.4698, 11.8402)
  line L234 (85.4698, 11.8402) -> (85.4698, 11.482)
  line L235 (85.4698, 11.482) -> (84.1903, 11.482)
  line L236 (84.1903, 11.482) -> (84.1903, 10.6694)
  spline S223 degree 2 poles (84.1903, 10.6694) (84.2644, 10.6793) (84.4077, 10.6867) (84.467, 10.6867) knots 0 0 0 1 2 2 2
  spline S224 degree 2 poles (84.467, 10.6867) (84.7016, 10.6867) (85.0252, 10.6101) (85.1734, 10.4965) knots 0 0 0 1 2 2 2
  spline S225 degree 2 poles (85.1734, 10.4965) (85.324, 10.3829) (85.4871, 10.037) (85.4871, 9.7604) knots 0 0 0 1 2 2 2
  line L237 (86.5813, 8.7922) -> (86.0922, 8.7922)
  line L238 (86.0922, 8.7922) -> (86.0922, 9.3751)
  line L239 (86.0922, 9.3751) -> (86.5813, 9.3751)
  line L240 (86.5813, 9.3751) -> (86.5813, 8.7922)
  spline S226 degree 2 poles (89.0933, 10.3162) (89.0933, 9.4961) (88.6166, 8.7279) (88.1201, 8.7279) knots 0 0 0 1 2 2 2
  spline S227 degree 2 poles (88.1201, 8.7279) (87.6162, 8.7279) (87.1444, 9.5109) (87.1444, 10.3137) knots 0 0 0 1 2 2 2
  spline S228 degree 2 poles (87.1444, 10.3137) (87.1444, 11.1387) (87.6212, 11.9019) (88.1201, 11.9019) knots 0 0 0 1 2 2 2
  spline S229 degree 2 poles (88.1201, 11.9019) (88.6215, 11.9019) (89.0933, 11.1115) (89.0933, 10.3162) knots 0 0 0 1 2 2 2
  spline S230 degree 2 poles (88.5696, 9.3874) (88.6289, 9.5381) (88.6783, 10.0025) (88.6783, 10.3162) knots 0 0 0 1 2 2 2
  spline S231 degree 2 poles (88.6783, 10.3162) (88.6783, 10.6299) (88.6289, 11.0917) (88.5672, 11.2474) knots 0 0 0 1 2 2 2
  spline S232 degree 2 poles (88.5672, 11.2474) (88.5054, 11.403) (88.2905, 11.5635) (88.1201, 11.5635) knots 0 0 0 1 2 2 2
  spline S233 degree 2 poles (88.1201, 11.5635) (87.9497, 11.5635) (87.7298, 11.403) (87.6656, 11.2424) knots 0 0 0 1 2 2 2
  spline S234 degree 2 poles (87.6656, 11.2424) (87.6039, 11.0868) (87.5594, 10.6126) (87.5594, 10.3137) knots 0 0 0 1 2 2 2
  spline S235 degree 2 poles (87.5594, 10.3137) (87.5594, 9.9926) (87.5989, 9.5628) (87.6632, 9.3948) knots 0 0 0 1 2 2 2
  spline S236 degree 2 poles (87.6632, 9.3948) (87.7224, 9.2368) (87.9423, 9.0663) (88.1201, 9.0663) knots 0 0 0 1 2 2 2
  spline S237 degree 2 poles (88.1201, 9.0663) (88.2881, 9.0663) (88.5079, 9.2269) (88.5696, 9.3874) knots 0 0 0 1 2 2 2
  spline S238 degree 2 poles (3.7765, 4.9791) (3.7765, 4.406) (3.2306, 3.7292) (2.8132, 3.7292) knots 0 0 0 1 2 2 2
  spline S239 degree 2 poles (2.8132, 3.7292) (2.6427, 3.7292) (2.3809, 3.8083) (2.245, 3.8898) knots 0 0 0 1 2 2 2
  line L241 (2.245, 3.8898) -> (2.245, 2.9314)
  line L242 (2.245, 2.9314) -> (1.8597, 2.9314)
  line L243 (1.8597, 2.9314) -> (1.8597, 6.0609)
  line L244 (1.8597, 6.0609) -> (2.245, 6.0609)
  line L245 (2.245, 6.0609) -> (2.245, 5.8214)
  spline S240 degree 2 poles (2.245, 5.8214) (2.3883, 5.9523) (2.7391, 6.1252) (2.9441, 6.1252) knots 0 0 0 1 2 2 2
  spline S241 degree 2 poles (2.9441, 6.1252) (3.3368, 6.1252) (3.7765, 5.5027) (3.7765, 4.9791) knots 0 0 0 1 2 2 2
  spline S242 degree 2 poles (3.3788, 4.9346) (3.3788, 5.3273) (3.1293, 5.7596) (2.8502, 5.7596) knots 0 0 0 1 2 2 2
  spline S243 degree 2 poles (2.8502, 5.7596) (2.6872, 5.7596) (2.3809, 5.6139) (2.245, 5.5003) knots 0 0 0 1 2 2 2
  line L246 (2.245, 5.5003) -> (2.245, 4.201)
  spline S244 degree 2 poles (2.245, 4.201) (2.3957, 4.1294) (2.6106, 4.0751) (2.7489, 4.0751) knots 0 0 0 1 2 2 2
  spline S245 degree 2 poles (2.7489, 4.0751) (3.0478, 4.0751) (3.3788, 4.5147) (3.3788, 4.9346) knots 0 0 0 1 2 2 2
  line L247 (4.5693, 3.7737) -> (4.184, 3.7737)
  line L248 (4.184, 3.7737) -> (4.184, 6.0609)
  line L249 (4.184, 6.0609) -> (4.5693, 6.0609)
  line L250 (4.5693, 6.0609) -> (4.5693, 3.7737)
  line L251 (4.5965, 6.4413) -> (4.1593, 6.4413)
  line L252 (4.1593, 6.4413) -> (4.1593, 6.8415)
  line L253 (4.1593, 6.8415) -> (4.5965, 6.8415)
  line L254 (4.5965, 6.8415) -> (4.5965, 6.4413)
  spline S246 degree 2 poles (5.8266, 3.7292) (5.5129, 3.7292) (5.1597, 4.0874) (5.1597, 4.4752) knots 0 0 0 1 2 2 2
  line L255 (5.1597, 4.4752) -> (5.1597, 5.7423)
  line L256 (5.1597, 5.7423) -> (4.9003, 5.7423)
  line L257 (4.9003, 5.7423) -> (4.9003, 6.0609)
  line L258 (4.9003, 6.0609) -> (5.1597, 6.0609)
  line L259 (5.1597, 6.0609) -> (5.1597, 6.718)
  line L260 (5.1597, 6.718) -> (5.545, 6.718)
  line L261 (5.545, 6.718) -> (5.545, 6.0609)
  line L262 (5.545, 6.0609) -> (6.2539, 6.0609)
  line L263 (6.2539, 6.0609) -> (6.2539, 5.7423)
  line L264 (6.2539, 5.7423) -> (5.545, 5.7423)
  line L265 (5.545, 5.7423) -> (5.545, 4.653)
  spline S247 degree 2 poles (5.545, 4.653) (5.545, 4.4801) (5.5573, 4.2899) (5.5993, 4.2084) knots 0 0 0 1 2 2 2
  spline S248 degree 2 poles (5.5993, 4.2084) (5.6339, 4.1368) (5.7895, 4.0652) (5.9229, 4.0652) knots 0 0 0 1 2 2 2
  spline S249 degree 2 poles (5.9229, 4.0652) (6.0168, 4.0652) (6.1921, 4.122) (6.2317, 4.1393) knots 0 0 0 1 2 2 2
  line L266 (6.2317, 4.1393) -> (6.2539, 4.1393)
  line L267 (6.2539, 4.1393) -> (6.2539, 3.7935)
  spline S250 degree 2 poles (6.2539, 3.7935) (6.1452, 3.7638) (5.9229, 3.7292) (5.8266, 3.7292) knots 0 0 0 1 2 2 2
  spline S251 degree 2 poles (7.4469, 3.7218) (7.2098, 3.7218) (6.817, 3.8676) (6.6763, 4.0158) knots 0 0 0 1 2 2 2
  spline S252 degree 2 poles (6.6763, 4.0158) (6.5355, 4.1615) (6.3799, 4.611) (6.3799, 4.9124) knots 0 0 0 1 2 2 2
  spline S253 degree 2 poles (6.3799, 4.9124) (6.3799, 5.2137) (6.5404, 5.6534) (6.6763, 5.8016) knots 0 0 0 1 2 2 2
  spline S254 degree 2 poles (6.6763, 5.8016) (6.8121, 5.9523) (7.2147, 6.1128) (7.4469, 6.1128) knots 0 0 0 1 2 2 2
  spline S255 degree 2 poles (7.4469, 6.1128) (7.6346, 6.1128) (7.9854, 6.0066) (8.1212, 5.9374) knots 0 0 0 1 2 2 2
  line L268 (8.1212, 5.9374) -> (8.1212, 5.5052)
  line L269 (8.1212, 5.5052) -> (8.099, 5.5052)
  spline S256 degree 2 poles (8.099, 5.5052) (8.057, 5.5398) (7.9286, 5.6287) (7.8372, 5.6756) knots 0 0 0 1 2 2 2
  spline S257 degree 2 poles (7.8372, 5.6756) (7.7557, 5.7151) (7.5383, 5.7769) (7.4395, 5.7769) knots 0 0 0 1 2 2 2
  spline S258 degree 2 poles (7.4395, 5.7769) (7.1406, 5.7769) (6.7775, 5.3249) (6.7775, 4.9124) knots 0 0 0 1 2 2 2